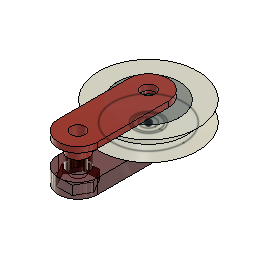
pulleys v7 (Autodesk Fusion 360 design; units mm, degrees)
Autodesk Fusion 360 part; units mm, degrees
sketch "Sketch1" plane through (0, 0, 0) normal (0, 0, 1) x (1, 0, 0) in component "608 Bearing"
  circle A0 centre (0, 0) radius 11
  circle A1 centre (0, 0) radius 4
  dimension "d10" = 22
  dimension "d11" = 8
  constraint coincident A0.centre A1.centre
  constraint concentric A0 A1
  measures "d10" diameter of A0
  measures "d11" diameter of A1
extrude "Extrude1" add sketch "Sketch1" along normal blind 7 makes body 1 in component "608 Bearing"
sketch "Sketch1 (2)" plane through (0, 0, 0) normal (0, 1, 0) x (1, 0, 0) in component "Wheel"
  line L0 (11, 0) -> (13.5, 0)
  line L1 (13.5, 0) -> (13.5, -7)
  line L2 (13.5, -7) -> (11, -7)
  line L3 (11, -7) -> (11, 0)
  line L4 (0, 0) -> (0, -16.6783)
  line L5 (13.5, -7) -> (17.5, -7)
  line L6 (17.5, -7) -> (13.5, -4.1992)
  line L7 (13.5, 0) -> (17.5, 0)
  line L8 (17.5, 0) -> (13.5, -2.8008)
  dimension "d1" = 2.5
  dimension "d2" = 7
  dimension "d6" = 22
  dimension "d7" = 4
  dimension "d46" = 35
  constraint horizontal L0
  constraint vertical L1
  constraint horizontal L2
  constraint vertical L3
  constraint coincident L4.start origin
  constraint vertical L4
  constraint perpendicular L1 L5
  constraint coincident L1 L6.end
  constraint perpendicular L1 L7
  constraint coincident L1 L8.end
  constraint vertical L5.end L7.end
  constraint equal L6 L8
  measures "d1" distance of L0.start L0.end
  measures "d2" distance of L0.start L2.end
  measures "d7" distance of L1.end L5.end
  measures "d46" angle of L5 L6
revolve "Revolve1" add sketch "Sketch1 (2)" angle 360 about axis through (0, 0, 0) along (0, 0, 1) separate body makes body 2 in component "Wheel"
sketch "Sketch1 (3)" plane through (0, 0, 0) normal (0, 0, 1) x (1, 0, 0) in component "Bracket"
  circle A0 centre (0, 0) radius 4
  line L0 (-7, 0) -> (-7, -25)
  arc A1 (-7, -25) -> (7, -25) centre (0, -25) ccw
  line L1 (7, -25) -> (7, 0)
  arc A2 (7, 0) -> (-7, 0) centre (0, 0) ccw
  line L2 (0, 0) -> (0, -25) construction
  circle A3 centre (0, -25) radius 2.5
  circle A4 centre (0, 0) radius 2.5
  circle A5 centre (0, 0) radius 5.5
  circle A6 centre (0, -25) radius 3.7
  dimension "d14" = 8
  dimension "d16" = 25
  dimension "d17" = 3
  dimension "d18" = 5
  dimension "d21" = 5
  dimension "d24" = 1.5
  dimension "d42" = 1.2
  constraint coincident A0.centre A2.centre
  constraint tangent L0 A1
  constraint tangent A1 L1
  constraint parallel L0 L1
  constraint tangent L1 A2
  constraint tangent L0 A2
  constraint vertical L2
  constraint concentric A1 A3
  constraint concentric A0 A4
  constraint concentric A3 A6
  measures "d14" diameter of A0
  measures "d16" distance of A0.centre A1.centre
  measures "d17" distance of A0 A2
  measures "d18" diameter of A3
  measures "d21" diameter of A4
  measures "d42" distance of A3 A6
extrude "Extrude1'" add sketch "Sketch1 (3)" against normal blind 2 from surface at -1 separate body contours A0 | L0 A1 L1 A2 | A5 | A6 makes body 3 in component "Bracket"
extrude "Extrude4" add sketch "Sketch1 (3)" against normal up to surface (1 mm away) contours A0 | A5 | A6 bodies 3 in component "Bracket"
extrude "Extrude5" add sketch "Sketch1 (3)" along normal blind 3.5 contours A0 | A6 bodies 3 in component "Bracket"
mirror "Mirror1" about plane through (0, 0, 3.5) normal (0, 0, 1) of bodies 3 makes body 4 in component "Bracket"
copy_body "Body->Comp1" bodies 4 removing the originals makes body 5 in component "BracketTop"
copy_body "Body->Comp2" bodies 3 removing the originals makes body 6 in component "BracketBottom"
combine "Combine1" operation cut target body 5 tool bodies 6 keep tools in component "BracketTop"
extrude "Extrude3" add 1 faces at (-5.0833, -9.055, -3) along direction (0, 0, -1) blind 3.175 on bodies 6 bodies 6 in component "BracketBottom"
sketch "Sketch1 (4)" plane through (0, 0, -6.175) normal (0, 0, -1) x (1, 0, 0) in component "BracketBottom"
  line L0 (-2.7929, 4.8375) -> (-5.5859, 0)
  line L1 (-5.5859, 0) -> (-2.7929, -4.8375)
  line L2 (-2.7929, -4.8375) -> (2.7929, -4.8375)
  line L3 (2.7929, -4.8375) -> (5.5859, 0)
  line L4 (5.5859, 0) -> (2.7929, 4.8375)
  line L5 (2.7929, 4.8375) -> (-2.7929, 4.8375)
  circle A0 centre (0, 0) radius 2.5
  circle A1 centre (0, 25) radius 2.5
  arc A2 (-7, 0) -> (7, 0) centre (0, 0) ccw
  line L6 (7, 0) -> (7, 25)
  arc A3 (7, 25) -> (-7, 25) centre (0, 25) ccw
  line L7 (-7, 25) -> (-7, 0)
  circle A4 centre (0, 0) radius 2.5
  circle A5 centre (0, 25) radius 2.5
  arc A6 (-7, 0) -> (7, 0) centre (0, 0) ccw
  line L8 (7, 0) -> (7, 25)
  arc A7 (7, 25) -> (-7, 25) centre (0, 25) ccw
  line L9 (-7, 25) -> (-7, 0)
  line L10 (2.7929, 20.1625) -> (5.5859, 25)
  line L11 (5.5859, 25) -> (2.7929, 29.8375)
  line L12 (2.7929, 29.8375) -> (-2.7929, 29.8375)
  line L13 (-2.7929, 29.8375) -> (-5.5859, 25)
  line L14 (-5.5859, 25) -> (-2.7929, 20.1625)
  line L15 (-2.7929, 20.1625) -> (2.7929, 20.1625)
  point P0 (0, 25)
  dimension "d37" = 9.675
  constraint coincident A0.centre A2.centre
  constraint horizontal L5
  constraint coincident P0 A1.centre
  constraint equal L5 L15
  constraint horizontal L15
  measures "d37" distance of L2 L5
extrude "Extrude2" [suppressed] in component "608 Bearing"
extrude "Extrude2'" cut sketch "Sketch1 (4)" against normal blind 3.175 contours L0 L1 L2 L3 L4 L5 | A0 A4 | L10 L11 L12 L13 L14 L15 bodies 6 in component "BracketBottom"
sketch "Sketch1 (5)" plane through (0, 0, 0) normal (0, 0, 1) x (1, 0, 0) in component "SingleBearingStandoff"
  circle A0 centre (0, 0) radius 2.5
  circle A1 centre (0, 0) radius 4.75
  circle A2 centre (0, 0) radius 4
  circle A3 centre (0, 0) radius 12.5
  dimension "d47" = 5
  dimension "d48" = 9.5
  dimension "d49" = 8
  dimension "d50" = 25
  constraint coincident A0.centre A1.centre
  constraint concentric A0 A2
  constraint concentric A1 A3
  measures "d47" diameter of A0
  measures "d48" diameter of A1
  measures "d49" diameter of A2
  measures "d50" diameter of A3
extrude "Extrude1''" add sketch "Sketch1 (5)" against normal blind 1 separate body contours A1 | A2 makes body 7 in component "SingleBearingStandoff"
extrude "Extrude2''" add sketch "Sketch1 (5)" against normal blind 2 from surface at -1 contours A1 | A2 | A3 bodies 7 in component "SingleBearingStandoff"
extrude "Extrude3'" add sketch "Sketch1 (5)" along normal blind 7 contours A2 bodies 7 in component "SingleBearingStandoff"
sketch "Sketch1 (6)" plane through (0, 0, 0) normal (0, 0, 1) x (1, 0, 0) in component "DoubleBearingStandoff"
  circle A0 centre (0, 0) radius 2.5
  circle A1 centre (0, 0) radius 5.5
  circle A2 centre (0, 0) radius 4
  circle A3 centre (0, 0) radius 12.5
  dimension "d47_1" = 5
  dimension "d49_1" = 8
  dimension "d50_1" = 25
  dimension "d61" = 1.5
  constraint coincident A0.centre A1.centre
  constraint concentric A0 A2
  constraint concentric A1 A3
  measures "d47_1" diameter of A0
  measures "d49_1" diameter of A2
  measures "d50_1" diameter of A3
  measures "d61" distance of A1 A2
extrude "Extrude1'''" add sketch "Sketch1 (6)" against normal blind 1 separate body contours A1 | A2 makes body 8 in component "DoubleBearingStandoff"
extrude "Extrude2'''" add sketch "Sketch1 (6)" against normal blind 2 from surface at -1 contours A1 | A2 | A3 bodies 8 in component "DoubleBearingStandoff"
extrude "Extrude3''" add sketch "Sketch1 (6)" along normal blind 15 contours A2 bodies 8 in component "DoubleBearingStandoff"
sketch "Sketch1 (7)" plane through (0, 0, 7) normal (0, 0, 1) x (-1, 0, 0) in component "Spacer"
  circle A0 centre (0, 0) radius 4
  circle A1 centre (0, 0) radius 11
  circle A2 centre (0, 0) radius 4
  circle A3 centre (0, 0) radius 5
  dimension "d59" = 8
  dimension "d60" = 1
  constraint coincident A0.centre A1.centre
  constraint concentric A2 A3
  measures "d59" diameter of A2
  measures "d60" distance of A2 A3
extrude "Extrude1''''" add sketch "Sketch1 (7)" along normal blind 1 separate body contours A3 makes body 9 in component "Spacer"
sketch "Sketch1 (8)" plane through (0, 0, 7) normal (0, 0, 1) x (-1, 0, 0) in component "Washer"
  circle A0 centre (0, 0) radius 4
  circle A1 centre (0, 0) radius 11
extrude "Extrude1'''''" add sketch "Sketch1 (5)" along normal blind 1 from surface at 7 separate body contours A1 | A2 makes body 10 in component "Washer"
component "608 Bearing" placed x (1, 0, 0) y (0, 1, 0) z (0, 0, 1) at (0, 0, 0)
component "Wheel" placed x (1, 0, 0) y (0, 1, 0) z (0, 0, 1) at (0, 0, 0)
component "Bracket" placed x (1, 0, 0) y (0, 1, 0) z (0, 0, 1) at (0, 0, 0)
component "SingleBearingStandoff" placed x (1, 0, 0) y (0, 1, 0) z (0, 0, 1) at (0, 0, 0)
component "DoubleBearingStandoff" placed x (1, 0, 0) y (0, 1, 0) z (0, 0, 1) at (0, 0, 0)
component "BracketTop" placed x (1, 0, 0) y (0, 1, 0) z (0, 0, 1) at (0, 0, 0) in component "Bracket"
component "BracketBottom" placed x (1, 0, 0) y (0, 1, 0) z (0, 0, 1) at (0, 0, 0) in component "Bracket"
component "Washer" placed x (1, 0, 0) y (0, 1, 0) z (0, 0, 1) at (0, 0, 0) in component "SingleBearingStandoff"
component "Spacer" placed x (1, 0, 0) y (0, 1, 0) z (0, 0, 1) at (0, 0, 0) in component "DoubleBearingStandoff"
equation "d37 = 0.375 in + 0.15 mm"
equation "d38 = -nutpocket"
equation "d40 = -nutpocket"
equation "d43 = nutpocket"
equation "nutpocket = 0.125 in"
equation "d56_1 = 7 mm * 2 + 1 mm"
named bodies: "Wheel", "608 Bearing", "BracketTop", "BracketBottom", "SingleBearingStandoff", "DoubleBearingStandoff", "Spacer", "Washer"
